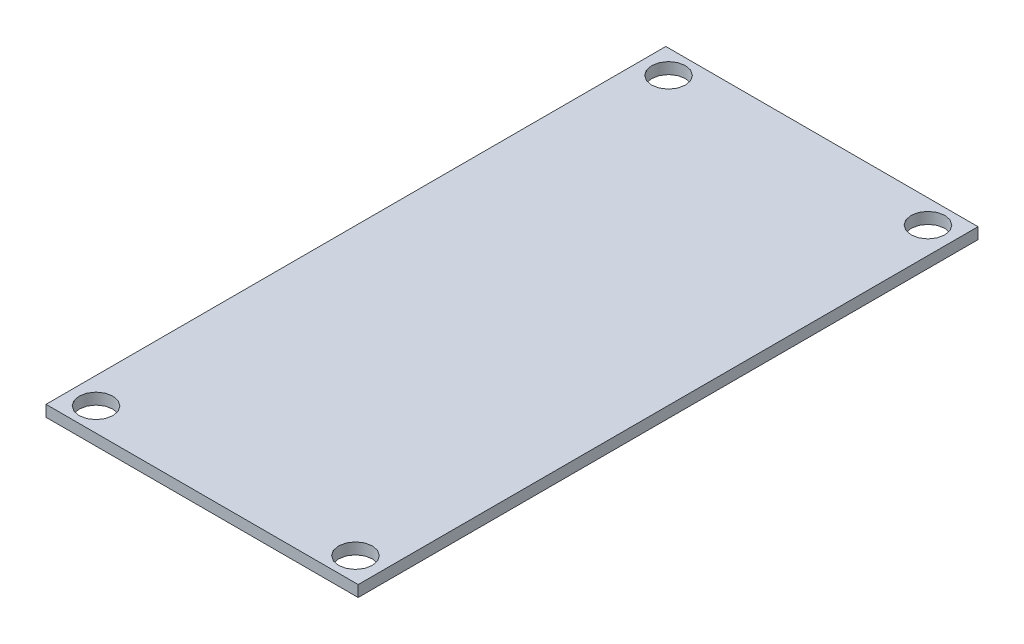
# Autodesk Inventor part: esp32_footprint
Saved by Autodesk Inventor 2019 (Build 230136000, 136)
## iProperties
Created: 2019-04-09
Part Number: esp32_footprint
Material: Generic
Document SubType Name: Modeling
Designer: jmc
Density: 1 g/cm^3
Appearance: Default
Author: jmc
Autodesk Inventor part; units mm, degrees
ref_plane "YZ Plane" through (0, 0, 0) normal (1, 0, 0) x (0, 1, 0)
ref_plane "XZ Plane" through (0, 0, 0) normal (0, 1, 0) x (-1, 0, 0)
ref_plane "XY Plane" through (0, 0, 0) normal (0, 0, 1) x (1, 0, 0)
sketch "Sketch1" plane through (0, 0, 0) normal (0, 1, 0) x (-1, 0, 0)
  line L0 (13.85, 27.5) -> (-13.85, 27.5)
  line L1 (-13.85, 27.5) -> (-13.85, -27.5)
  line L2 (-13.85, -27.5) -> (13.85, -27.5)
  line L3 (13.85, -27.5) -> (13.85, 27.5)
  line L4 (13.85, 27.5) -> (-13.85, -27.5) construction
  line L5 (-13.85, 27.5) -> (13.85, -27.5) construction
  line L6 (0, 27.5) -> (0, -27.5) construction
  line L7 (13.85, 0) -> (-13.85, 0) construction
  circle A0 centre (11.51, 25.4) radius 1.5
  circle A1 centre (11.51, -25.4) radius 1.5
  circle A2 centre (-11.51, 25.4) radius 1.5
  circle A3 centre (-11.51, -25.4) radius 1.5
  point P0 (0, 0)
  dimension "d0" = 27.7
  dimension "d1" = 55
  dimension "d2" = 3
  dimension "d3" = 2.34
  dimension "d4" = 2.1
  constraints: 16 end point, 6 midpoint, 4 centre point, 3 symmetric about line, 2 parallel, 1 horizontal, 1 perpendicular, 3 other
  measures "d0" distance of L2.end L1.end
  measures "d1" distance of L1.end L0.end
  measures "d2" diameter of A0
  measures "d3" distance from line of L3 A0.centre
  measures "d4" distance from line of L0 A0.centre
extrude "Extrusion1" add sketch "Sketch1" along normal blind 1
body "Solid1"
